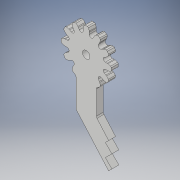
# Autodesk Inventor part: Part21
Saved by Autodesk Inventor 2019.2 (Build 232265000, 265)
## iProperties
Created: 2019-04-05
Part Number: Part21
Material: Generic
Document SubType Name: Modeling
Designer: richard.girt
Mass: 1.20236 g
Surface Area: 13.08 cm^2
Volume: 1.20236 cm^3
Density: 1 g/cm^3
Appearance: Default
Author: richard.girt
Autodesk Inventor part; units mm, degrees
ref_plane "YZ Plane" through (0, 0, 0) normal (1, 0, 0) x (0, 1, 0)
ref_plane "XZ Plane" through (0, 0, 0) normal (0, 1, 0) x (-1, 0, 0)
ref_plane "XY Plane" through (0, 0, 0) normal (0, 0, 1) x (1, 0, 0)
sketch "Sketch1" plane through (0, 0, 0) normal (0, 0, 1) x (1, 0, 0)
  circle A0 centre (0, 0) radius 1.5
  line L0 (10.3186, -34.6057) -> (9, -35.9244)
  line L1 (9, -35.9244) -> (-3.8225, -21.2975)
  arc A1 (-4.0704, -20.6384) -> (-3.8225, -21.2975) centre (-3.0704, -20.6384) ccw
  line L2 (-4.0704, -20.6384) -> (-4.0704, -9.8676)
  line L3 (4.0704, -9.8676) -> (4.0704, -19.3318)
  arc A2 (4.0704, -19.3318) -> (4.3183, -19.9909) centre (5.0704, -19.3318) ccw
  line L4 (4.3183, -19.9909) -> (9, -25.3753)
  line L5 (9, -25.3753) -> (7.6814, -26.694)
  line L6 (7.6814, -26.694) -> (10.3186, -29.3312)
  line L7 (10.3186, -29.3312) -> (7.6814, -31.9685)
  line L8 (7.6814, -31.9685) -> (10.3186, -34.6057)
  arc A3 (-0.8823, 9.7494) -> (-1.2074, 8.7514) centre (2.3891, 8.1317) ccw
  arc A4 (-0.4353, 10.0808) -> (-0.8823, 9.7494) centre (-0.4113, 9.5814) ccw
  arc A5 (-1.1882, 8.8542) -> (-1.2341, 8.4178) centre (0.8597, 8.4178) ccw
  line L9 (-1.2341, 8.4178) -> (-1.2341, 7.6771)
  arc A6 (-1.8441, 6.8822) -> (-1.2341, 7.6771) centre (-2.0571, 7.6771) ccw
  arc A7 (1.2074, 8.7514) -> (0.8823, 9.7494) centre (-2.3891, 8.1317) ccw
  arc A8 (0.8823, 9.7494) -> (0.4353, 10.0808) centre (0.4113, 9.5814) ccw
  arc A9 (1.2341, 8.4178) -> (1.2074, 8.7514) centre (-0.8597, 8.4178) ccw
  line L10 (1.2341, 8.4178) -> (1.2341, 7.6771)
  arc A10 (1.2341, 7.6771) -> (1.8441, 6.8822) centre (2.0571, 7.6771) ccw
  line L11 (-0.4353, 10.0808) -> (0.4353, 10.0808)
  arc A11 (-5.6388, 8.0021) -> (-5.4561, 7.0738) centre (-1.9968, 8.2368) ccw
  arc A12 (-5.4174, 8.5126) -> (-5.6388, 8.0021) centre (-5.1469, 8.092) ccw
  arc A13 (-5.4561, 7.0738) -> (-5.2777, 6.673) centre (-3.4644, 7.7199) ccw
  line L12 (-5.2777, 6.673) -> (-4.9074, 6.0315)
  arc A14 (-5.0381, 5.0381) -> (-4.9074, 6.0315) centre (-5.62, 5.62) ccw
  arc A15 (-3.33, 8.1826) -> (-4.1107, 8.8844) centre (-6.1349, 5.8477) ccw
  arc A16 (-4.1107, 8.8844) -> (-4.6634, 8.9479) centre (-4.4345, 8.5034) ccw
  arc A17 (-3.1401, 7.9071) -> (-3.3981, 8.262) centre (-4.9535, 6.8602) ccw
  line L13 (-3.1401, 7.9071) -> (-2.7698, 7.2656)
  arc A18 (-2.7698, 7.2656) -> (-1.8441, 6.8822) centre (-2.0571, 7.6771) ccw
  line L14 (-5.4174, 8.5126) -> (-4.6634, 8.9479)
  arc A19 (-8.8844, 4.1107) -> (-8.262, 3.3981) centre (-5.8477, 6.1349) ccw
  arc A20 (-8.9479, 4.6634) -> (-8.8844, 4.1107) centre (-8.5034, 4.4345) ccw
  arc A21 (-8.262, 3.3981) -> (-7.9071, 3.1401) centre (-6.8602, 4.9535) ccw
  line L15 (-7.9071, 3.1401) -> (-7.2656, 2.7698)
  arc A22 (-6.8822, 1.8441) -> (-7.2656, 2.7698) centre (-7.6771, 2.0571) ccw
  arc A23 (-6.9752, 5.4213) -> (-8.0021, 5.6388) centre (-8.2368, 1.9968) ccw
  arc A24 (-8.0021, 5.6388) -> (-8.5126, 5.4174) centre (-8.092, 5.1469) ccw
  arc A25 (-6.673, 5.2777) -> (-7.0738, 5.4561) centre (-7.7199, 3.4644) ccw
  line L16 (-6.673, 5.2777) -> (-6.0315, 4.9074)
  arc A26 (-6.0315, 4.9074) -> (-5.0381, 5.0381) centre (-5.62, 5.62) ccw
  line L17 (-8.9479, 4.6634) -> (-8.5126, 5.4174)
  arc A27 (-9.7494, -0.8823) -> (-8.8542, -1.1882) centre (-8.1317, 2.3891) ccw
  arc A28 (-10.0808, -0.4353) -> (-9.7494, -0.8823) centre (-9.5814, -0.4113) ccw
  arc A29 (-8.8542, -1.1882) -> (-8.4178, -1.2341) centre (-8.4178, 0.8597) ccw
  line L18 (-8.4178, -1.2341) -> (-7.6771, -1.2341)
  arc A30 (-6.8822, -1.8441) -> (-7.6771, -1.2341) centre (-7.6771, -2.0571) ccw
  arc A31 (-8.7514, 1.2074) -> (-9.7494, 0.8823) centre (-8.1317, -2.3891) ccw
  arc A32 (-9.7494, 0.8823) -> (-10.0808, 0.4353) centre (-9.5814, 0.4113) ccw
  arc A33 (-8.4178, 1.2341) -> (-8.7514, 1.2074) centre (-8.4178, -0.8597) ccw
  line L19 (-8.4178, 1.2341) -> (-7.6771, 1.2341)
  arc A34 (-7.6771, 1.2341) -> (-6.8822, 1.8441) centre (-7.6771, 2.0571) ccw
  line L20 (-10.0808, -0.4353) -> (-10.0808, 0.4353)
  arc A35 (-8.0021, -5.6388) -> (-6.9752, -5.4213) centre (-8.2368, -1.9968) ccw
  arc A36 (-8.5126, -5.4174) -> (-8.0021, -5.6388) centre (-8.092, -5.1469) ccw
  arc A37 (-7.0738, -5.4561) -> (-6.673, -5.2777) centre (-7.7199, -3.4644) ccw
  line L21 (-6.673, -5.2777) -> (-6.0315, -4.9074)
  arc A38 (-5.0381, -5.0381) -> (-6.0315, -4.9074) centre (-5.62, -5.62) ccw
  arc A39 (-8.1826, -3.33) -> (-8.8844, -4.1107) centre (-5.8477, -6.1349) ccw
  arc A40 (-8.8844, -4.1107) -> (-8.9479, -4.6634) centre (-8.5034, -4.4345) ccw
  arc A41 (-7.9071, -3.1401) -> (-8.1826, -3.33) centre (-6.8602, -4.9535) ccw
  line L22 (-7.9071, -3.1401) -> (-7.2656, -2.7698)
  arc A42 (-7.2656, -2.7698) -> (-6.8822, -1.8441) centre (-7.6771, -2.0571) ccw
  line L23 (-8.5126, -5.4174) -> (-8.9479, -4.6634)
  arc A43 (-5.4213, -6.9752) -> (-5.6388, -8.0021) centre (-1.9968, -8.2368) ccw
  arc A44 (-5.6388, -8.0021) -> (-5.4174, -8.5126) centre (-5.1469, -8.092) ccw
  arc A45 (-5.2777, -6.673) -> (-5.4213, -6.9752) centre (-3.4644, -7.7199) ccw
  line L24 (-5.2777, -6.673) -> (-4.9074, -6.0315)
  arc A46 (-4.9074, -6.0315) -> (-5.0381, -5.0381) centre (-5.62, -5.62) ccw
  line L25 (-4.5704, -9.0016) -> (-5.4174, -8.5126)
  arc A47 (-4.0704, -9.8676) -> (-4.5704, -9.0016) centre (-5.0704, -9.8676) ccw
  arc A48 (5.6388, -8.0021) -> (5.4213, -6.9752) centre (1.9968, -8.2368) ccw
  arc A49 (5.4174, -8.5126) -> (5.6388, -8.0021) centre (5.1469, -8.092) ccw
  arc A50 (5.4213, -6.9752) -> (5.2777, -6.673) centre (3.4644, -7.7199) ccw
  line L26 (5.2777, -6.673) -> (4.9074, -6.0315)
  arc A51 (5.0381, -5.0381) -> (4.9074, -6.0315) centre (5.62, -5.62) ccw
  line L27 (5.4174, -8.5126) -> (4.5704, -9.0016)
  arc A52 (4.5704, -9.0016) -> (4.0704, -9.8676) centre (5.0704, -9.8676) ccw
  arc A53 (8.8844, -4.1107) -> (8.1826, -3.33) centre (5.8477, -6.1349) ccw
  arc A54 (8.9479, -4.6634) -> (8.8844, -4.1107) centre (8.5034, -4.4345) ccw
  arc A55 (8.1826, -3.33) -> (7.9071, -3.1401) centre (6.8602, -4.9535) ccw
  line L28 (7.9071, -3.1401) -> (7.2656, -2.7698)
  arc A56 (6.8822, -1.8441) -> (7.2656, -2.7698) centre (7.6771, -2.0571) ccw
  arc A57 (7.0738, -5.4561) -> (8.0021, -5.6388) centre (8.2368, -1.9968) ccw
  arc A58 (8.0021, -5.6388) -> (8.5126, -5.4174) centre (8.092, -5.1469) ccw
  arc A59 (6.673, -5.2777) -> (7.0738, -5.4561) centre (7.7199, -3.4644) ccw
  line L29 (6.673, -5.2777) -> (6.0315, -4.9074)
  arc A60 (6.0315, -4.9074) -> (5.0381, -5.0381) centre (5.62, -5.62) ccw
  line L30 (8.9479, -4.6634) -> (8.5126, -5.4174)
  arc A61 (9.7494, 0.8823) -> (8.7514, 1.2074) centre (8.1317, -2.3891) ccw
  arc A62 (10.0808, 0.4353) -> (9.7494, 0.8823) centre (9.5814, 0.4113) ccw
  arc A63 (8.7514, 1.2074) -> (8.4178, 1.2341) centre (8.4178, -0.8597) ccw
  line L31 (8.4178, 1.2341) -> (7.6771, 1.2341)
  arc A64 (6.8822, 1.8441) -> (7.6771, 1.2341) centre (7.6771, 2.0571) ccw
  arc A65 (8.8542, -1.1882) -> (9.7494, -0.8823) centre (8.1317, 2.3891) ccw
  arc A66 (9.7494, -0.8823) -> (10.0808, -0.4353) centre (9.5814, -0.4113) ccw
  arc A67 (8.4178, -1.2341) -> (8.8542, -1.1882) centre (8.4178, 0.8597) ccw
  line L32 (8.4178, -1.2341) -> (7.6771, -1.2341)
  arc A68 (7.6771, -1.2341) -> (6.8822, -1.8441) centre (7.6771, -2.0571) ccw
  line L33 (10.0808, 0.4353) -> (10.0808, -0.4353)
  arc A69 (8.0021, 5.6388) -> (7.0738, 5.4561) centre (8.2368, 1.9968) ccw
  arc A70 (8.5126, 5.4174) -> (8.0021, 5.6388) centre (8.092, 5.1469) ccw
  arc A71 (7.0738, 5.4561) -> (6.673, 5.2777) centre (7.7199, 3.4644) ccw
  line L34 (6.673, 5.2777) -> (6.0315, 4.9074)
  arc A72 (5.0381, 5.0381) -> (6.0315, 4.9074) centre (5.62, 5.62) ccw
  arc A73 (8.262, 3.3981) -> (8.8844, 4.1107) centre (5.8477, 6.1349) ccw
  arc A74 (8.8844, 4.1107) -> (8.9479, 4.6634) centre (8.5034, 4.4345) ccw
  arc A75 (7.9071, 3.1401) -> (8.262, 3.3981) centre (6.8602, 4.9535) ccw
  line L35 (7.9071, 3.1401) -> (7.2656, 2.7698)
  arc A76 (7.2656, 2.7698) -> (6.8822, 1.8441) centre (7.6771, 2.0571) ccw
  line L36 (8.5126, 5.4174) -> (8.9479, 4.6634)
  arc A77 (4.1107, 8.8844) -> (3.3981, 8.262) centre (6.1349, 5.8477) ccw
  arc A78 (4.6634, 8.9479) -> (4.1107, 8.8844) centre (4.4345, 8.5034) ccw
  arc A79 (3.3981, 8.262) -> (3.1401, 7.9071) centre (4.9535, 6.8602) ccw
  line L37 (3.1401, 7.9071) -> (2.7698, 7.2656)
  arc A80 (1.8441, 6.8822) -> (2.7698, 7.2656) centre (2.0571, 7.6771) ccw
  arc A81 (5.4213, 6.9752) -> (5.6388, 8.0021) centre (1.9968, 8.2368) ccw
  arc A82 (5.6388, 8.0021) -> (5.4174, 8.5126) centre (5.1469, 8.092) ccw
  arc A83 (5.2777, 6.673) -> (5.4213, 6.9752) centre (3.4644, 7.7199) ccw
  line L38 (5.2777, 6.673) -> (4.9074, 6.0315)
  arc A84 (4.9074, 6.0315) -> (5.0381, 5.0381) centre (5.62, 5.62) ccw
  line L39 (4.6634, 8.9479) -> (5.4174, 8.5126)
  point P0 (0, 0)
  dimension "d0" = 3
  constraints: 208 point on circle, 85 centre point, 80 end point
  measures "d0" diameter of A0
extrude "Extrusion1" add sketch "Sketch1" along normal mid plane 2.8 contours A0 | L0 L1 A1 L2 A47 L25 A44 A43 A45 L24 A46 A38 L21 A37 A35 A36 L23 A40 A39 A41 L22 A42 A30 L18 A29 A27 A28 L20 A32 A31 A33 L19 A34 A22 L15 A21 A19 A20 L17 A24 A23 A25 L16 A26 A14 L12 A13 A11 A12 L14 A16 A15 A17 L13 A18 A6 L9 A5 A3 A4 L11 A8 A7 A9 L10 A10 A80 L37 A79 A77 A78 L39 A82 A81 A83 L38 A84 A72 L34 A71 A69 A70 L36 A74 A73 A75 L35 A76 A64 L31 A63 A61 A62 L33 A66 A65 A67 L32 A68 A56 L28 A55 A53 A54 L30 A58 A57 A59 L29 A60 A51 L26 A50 A48 A49 L27 A52 L3 A2 L4 L5 L6 L7 L8
extrude "Extrusion2" cut sketch "Sketch1" along normal through all both and the other way through all contours A0
body "Solid1"
